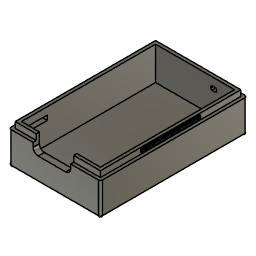
SlimCase-502030-FDM v6 (Autodesk Fusion 360 design; units mm, degrees)
Autodesk Fusion 360 part; units mm, degrees
sketch "Sketch1" plane through (0, 0, 0) normal (0, 0, 1) x (1, 0, 0)
  line L0 (10.1, -17.15) -> (-10.1, -17.15)
  line L1 (-10.1, -17.15) -> (-10.1, 17.15)
  line L2 (-10.1, 17.15) -> (10.1, 17.15)
  line L3 (10.1, 17.15) -> (10.1, -17.15)
  line L4 (10.1, -17.15) -> (-10.1, 17.15) construction
  line L5 (-10.1, -17.15) -> (10.1, 17.15) construction
  line L6 (11.7, 18.75) -> (-11.7, 18.75)
  line L7 (-11.7, 18.75) -> (-11.7, -18.75)
  line L8 (-11.7, -18.75) -> (11.7, -18.75)
  line L9 (11.7, -18.75) -> (11.7, 18.75)
  line L10 (11.7, 18.75) -> (-11.7, -18.75) construction
  line L11 (-11.7, 18.75) -> (11.7, -18.75) construction
  dimension "d1" = 20.2
  dimension "d2" = 34.3
  dimension "d4" = 1.6
  dimension "d5" = 1.6
  constraint horizontal L0
  constraint perpendicular L0 L1
  constraint parallel L0 L2
  constraint parallel L1 L3
  constraint coincident L4 origin
  constraint coincident L5 origin
  constraint horizontal L6
  constraint perpendicular L6 L7
  constraint parallel L6 L8
  constraint parallel L7 L9
  constraint coincident L10 origin
  constraint coincident L11 origin
  measures "d1" distance of L1.end L2.end
  measures "d2" distance of L0.end L1.end
  measures "d4" distance of L2 L6
  measures "d5" distance of L1 L7
extrude "Extrude1" add sketch "Sketch1" along normal blind 7
sketch "Sketch2" plane through (0, 0, 0) normal (0, 0, -1) x (1, 0, 0)
  line L0 (10.1, -17.15) -> (-10.1, -17.15)
  line L1 (-10.1, -17.15) -> (-10.1, 17.15)
  line L2 (-10.1, 17.15) -> (10.1, 17.15)
  line L3 (10.1, 17.15) -> (10.1, -17.15)
  line L4 (11.7, -18.75) -> (11.7, 18.75)
  line L5 (11.7, 18.75) -> (-11.7, 18.75)
  line L6 (-11.7, 18.75) -> (-11.7, -18.75)
  line L7 (-11.7, -18.75) -> (11.7, -18.75)
  line L8 (-11.7, 18.75) -> (11.7, 18.75)
  line L9 (11.7, 18.75) -> (11.7, -18.75)
  line L10 (11.7, -18.75) -> (-11.7, -18.75)
  line L11 (-11.7, -18.75) -> (-11.7, 18.75)
  constraint horizontal L8
  constraint vertical L9
  constraint horizontal L10
  constraint vertical L11
  constraint coincident L4.start L7.end
  constraint coincident L5.end L6.start
extrude "Extrude2" add sketch "Sketch2" along normal blind 1.4 contours L0 L1 L2 L3 | L4 L5 L6 L7 L8 L9 L10 L11
sketch "Sketch3" plane through (0, -18.75, 0) normal (0, -1, 0) x (1, 0, 0)
  line L0 (11.7, -1.4) -> (11.7, 7)
  line L1 (11.7, 7) -> (-11.7, 7)
  line L2 (-11.7, 7) -> (-11.7, -1.4)
  line L3 (-11.7, -1.4) -> (11.7, -1.4)
  line L4 (-5.52, 7) -> (4.08, 7)
  line L5 (4.08, 7) -> (4.08, 4.6)
  line L6 (4.08, 4.6) -> (-5.52, 4.6)
  line L7 (-5.52, 4.6) -> (-5.52, 7)
  dimension "d10" = 6
  dimension "d11" = 6.18
  dimension "d14" = 9.6
  constraint horizontal L4
  constraint vertical L5
  constraint horizontal L6
  constraint vertical L7
  constraint coincident L1 L4.start
  measures "d10" distance of L3 L6
  measures "d11" distance of L2 L7
  measures "d14" distance of L4.start L4.end
extrude "Extrude3" cut sketch "Sketch3" against normal up to surface (1.6 mm away) contours L1 L4 L5 L6 L7
fillet "Fillet1" radius 1.3 2 edges at (-5.52, -17.95, 4.6) (4.08, -17.95, 4.6)
sketch "Sketch4" plane through (-11.7, 0, 0) normal (-1, 0, 0) x (0, -1, 0)
  line L0 (18.75, -1.4) -> (18.75, 7)
  line L1 (18.75, 7) -> (-18.75, 7)
  line L2 (-18.75, 7) -> (-18.75, -1.4)
  line L3 (-18.75, -1.4) -> (18.75, -1.4)
  line L4 (10.55, 6.65) -> (15.55, 6.65)
  line L5 (15.55, 6.65) -> (15.55, 5.45)
  line L6 (15.55, 5.45) -> (10.55, 5.45)
  line L7 (10.55, 5.45) -> (10.55, 6.65)
  dimension "d17" = 3.2
  dimension "d18" = 5
  dimension "d19" = 1.2
  dimension "d22" = 0.35
  constraint horizontal L4
  constraint vertical L5
  constraint horizontal L6
  constraint vertical L7
  measures "d17" distance of L0 L5
  measures "d18" distance of L4.start L4.end
  measures "d19" distance of L4.start L6.end
  measures "d22" distance of L1 L4
extrude "Extrude4" cut sketch "Sketch4" against normal up to surface (1.6 mm away) contours L4 L5 L6 L7
fillet "Fillet2" radius 0.15 4 edges at (-11.7, -13.05, 5.45) (-11.7, -10.55, 6.05) (-11.7, -13.05, 6.65) (-11.7, -15.55, 6.05)
sketch "Sketch5" plane through (0, 0, 7) normal (0, 0, 1) x (-1, 0, 0)
  line L0 (-4.08, 17.15) -> (-4.08, 18.75)
  line L1 (-4.08, 18.75) -> (-11.7, 18.75)
  line L2 (-11.7, 18.75) -> (-11.7, -18.75)
  line L3 (-11.7, -18.75) -> (11.7, -18.75)
  line L4 (11.7, -18.75) -> (11.7, 18.75)
  line L5 (11.7, 18.75) -> (5.52, 18.75)
  line L6 (5.52, 18.75) -> (5.52, 17.15)
  line L7 (5.52, 17.15) -> (10.1, 17.15)
  line L8 (10.1, 17.15) -> (10.1, -17.15)
  line L9 (10.1, -17.15) -> (-10.1, -17.15)
  line L10 (-10.1, -17.15) -> (-10.1, 17.15)
  line L11 (-10.1, 17.15) -> (-4.08, 17.15)
  line L12 (10.9, -17.95) -> (-10.9, -17.95)
  line L13 (-10.9, -17.95) -> (-10.9, 17.95)
  line L14 (-10.9, 17.95) -> (10.9, 17.95)
  line L15 (10.9, 17.95) -> (10.9, -17.95)
  dimension "d26" = 0.8
  dimension "d27" = 0.8
  dimension "d28" = 0.8
  dimension "d29" = 0.8
  constraint horizontal L12
  constraint vertical L13
  constraint horizontal L14
  constraint vertical L15
  measures "d26" distance of L8 L15
  measures "d27" distance of L7 L14
  measures "d28" distance of L10 L13
  measures "d29" distance of L9 L12
extrude "Extrude5" add sketch "Sketch5" along normal blind 1.5 contours L0 L6 L7 L8 L9 L10 L11 L12 L13 L14 L15
sketch "Sketch7" plane through (10.9, 0, 0) normal (1, 0, 0) x (0, 1, 0)
  line L0 (-17.95, 7) -> (17.95, 7)
  line L1 (17.95, 7) -> (17.95, 8.5)
  line L2 (17.95, 8.5) -> (-17.95, 8.5)
  line L3 (-17.95, 8.5) -> (-17.95, 7)
  line L4 (-17.95, 8.5) -> (17.95, 7) construction
  line L5 (17.95, 8.5) -> (-17.95, 7) construction
  line L6 (0, 7.75) -> (-14.5, 7.75) construction
  line L7 (7.5, 7.45) -> (-7.5, 7.45)
  line L8 (-7.5, 7.45) -> (-7.5, 8.05)
  line L9 (-7.5, 8.05) -> (7.5, 8.05)
  line L10 (7.5, 8.05) -> (7.5, 7.45)
  line L11 (7.5, 7.45) -> (-7.5, 8.05) construction
  line L12 (-7.5, 7.45) -> (7.5, 8.05) construction
  point P0 (0, 7.75)
  dimension "d32" = 15
  dimension "d33" = 0.6
  constraint coincident L2.end L3.start
  constraint coincident L0.end L1.start
  constraint coincident L1.end L2.start
  constraint coincident L0.start L3.end
  constraint midpoint L4 P0
  constraint parallel L0 L6
  constraint horizontal L7
  constraint perpendicular L7 L8
  constraint parallel L7 L9
  constraint parallel L8 L10
  constraint coincident L11 P0
  constraint coincident L12 P0
  constraint coincident P0 L6.start
  measures "d32" distance of L8.end L9.end
  measures "d33" distance of L7.start L9.end
ref_plane "WorkPlane1" through (0, 0, 7.75) normal (1, 0, 0) x (0, 1, 0)
extrude "Extrude6" cut sketch "Sketch7" against normal blind 0.45 contours L7 L8 L9 L10
fillet "Fillet5" radius 0.2 4 edges at (10.675, -7.5, 7.45) (10.675, -7.5, 8.05) (10.675, 7.5, 7.45) (10.675, 7.5, 8.05)
fillet "Fillet6" radius 0.2 8 edges at (10.9, -7.4414, 7.5086) (10.9, 0, 7.45) (10.9, 7.4414, 7.5086) (10.9, 7.5, 7.75) (10.9, 7.4414, 7.9914) (10.9, 0, 8.05) (10.9, -7.4414, 7.9914) (10.9, -7.5, 7.75)
mirror "Mirror2" about plane through (0, 0, 7.75) normal (1, 0, 0) of "Extrude6"
fillet "Fillet7" radius 0.2 4 edges at (-10.675, 7.5, 7.45) (-10.675, 7.5, 8.05) (-10.675, -7.5, 7.45) (-10.675, -7.5, 8.05)
fillet "Fillet8" radius 0.2 8 edges at (-10.9, -7.4414, 7.9914) (-10.9, -7.5, 7.75) (-10.9, -7.4414, 7.5086) (-10.9, 0, 7.45) (-10.9, 7.4414, 7.5086) (-10.9, 7.5, 7.75) (-10.9, 7.4414, 7.9914) (-10.9, 0, 8.05)
fillet "Fillet9" radius 0.5 8 edges at (-11.7, 18.75, 2.8) (-11.7, -18.75, 2.8) (-11.7, 0, -1.4) (0, -18.75, -1.4) (11.7, -18.75, 2.8) (11.7, 0, -1.4) (11.7, 18.75, 2.8) (0, 18.75, -1.4)
sketch "Sketch8" plane through (0, 17.15, 0) normal (0, -1, 0) x (1, 0, 0)
  line L0 (-10.1, 0) -> (10.1, 0)
  line L1 (10.1, 0) -> (10.1, 8.5)
  line L2 (10.1, 8.5) -> (-10.1, 8.5)
  line L3 (-10.1, 8.5) -> (-10.1, 0)
  line L4 (4, 6.5) -> (5.5, 6.5)
  line L5 (5.5, 6.5) -> (5.5, 5.5)
  line L6 (5.5, 5.5) -> (4, 5.5)
  line L7 (4, 5.5) -> (4, 6.5)
  dimension "d55" = 4.6
  dimension "d56" = 1
  dimension "d57" = 1.5
  dimension "d58" = 2
  constraint horizontal L4
  constraint vertical L5
  constraint horizontal L6
  constraint vertical L7
  measures "d55" distance of L1 L5
  measures "d56" distance of L4.start L6.end
  measures "d57" distance of L5.end L6.end
  measures "d58" distance of L2 L4
extrude "Extrude7" cut sketch "Sketch8" against normal up to surface (1.6 mm away) contours L4 L5 L6 L7
fillet "Fillet10" radius 0.3 4 edges at (5.5, 17.95, 5.5) (5.5, 17.95, 6.5) (4, 17.95, 6.5) (4, 17.95, 5.5)
equation "case_thickness = 1.6 mm"
equation "d4 = case_thickness"
equation "d5 = case_thickness"
equation "d8 = case_thickness - 0.2 mm"
equation "d11 = 4.58 mm + case_thickness"
equation "lock_rim = 0.8 mm"
equation "d26 = lock_rim"
equation "d27 = lock_rim"
equation "d28 = lock_rim"
equation "d29 = lock_rim"
equation "d43 = clip_roundness"
equation "d45 = clip_roundness"
equation "clip_roundness = 0.2 mm"
equation "d50 = clip_roundness"
equation "d52 = clip_roundness"
